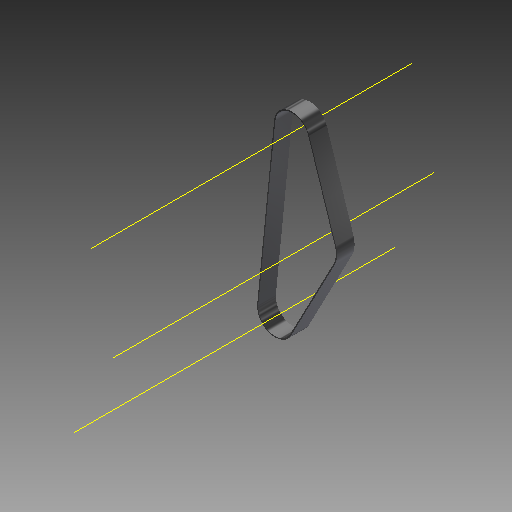
# Autodesk Inventor part: Synchronous Belt
Saved by Autodesk Inventor 2019.4 (Build 234330000, 330)
## iProperties
Created: 2020-01-06
Part Number: Synchronous Belt
Material: Rubber
Document SubType Name: Modeling
Designer: admin
Density: 1 g/cm^3
Appearance: Rubber - Black - Version 1.1
CustomPartVersion: 1
Author: admin
Autodesk Inventor part; units mm, degrees
ref_plane "YZ Plane" through (0, 0, 0) normal (1, 0, 0) x (0, 1, 0)
ref_plane "XZ Plane" through (0, 0, 0) normal (0, 1, 0) x (-1, 0, 0)
ref_plane "XY Plane" through (0, 0, 0) normal (0, 0, 1) x (1, 0, 0)
sketch "Sketch Path" plane through (0, 0, 0) normal (0, 0, 1) x (1, 0, 0)
  arc A0 (-17.1486, -148.689) -> (12.7796, -157.6858) centre (-1.314, -150.2918) ccw
  arc A1 (29.2855, 7.4127) -> (-1.6838, 4.0918) centre (14.1508, 2.489) ccw
  arc A2 (52.2256, -82.4982) -> (53.5269, -67.101) centre (34.6085, -73.2557) ccw
  line L0 (52.2256, -82.4982) -> (12.7796, -157.6858)
  line L1 (-17.1486, -148.689) -> (-1.6838, 4.0918)
  line L2 (29.2855, 7.4127) -> (53.5269, -67.101)
  constraints: 6 end point, 6 point on circle, 3 centre point
ref_plane "Cross Section Plane" through (12.7796, -157.6858, 0) normal (0.4645795, 0.8855314, 0) x (0, 0, 1)
ref_plane "Work Plane2" through (-1.314, -150.2918, 0) normal (-1, 0, 0) x (0, 0, 1)
ref_plane "Work Plane3" through (14.1508, 2.489, 0) normal (-0.3935975, -0.9192829, 0) x (0, 0, 1)
ref_plane "Work Plane4" through (34.6085, -73.2557, 0) normal (-0.1587052, 0.987326, 0) x (0, 0, 1)
sketch "Cross Section" plane through (12.7796, -157.6858, 0) normal (0.4645795, 0.8855314, 0) x (0, 0, 1)
  line L0 (-8, 0.5) -> (8, 0.5)
  line L1 (8, 0.5) -> (8, -0.5)
  line L2 (8, -0.5) -> (-8, -0.5)
  line L3 (-8, -0.5) -> (-8, 0.5)
  line L4 (-8, 0) -> (8, 0) construction
  point P0 (0, 0)
  point P1 (0, 0)
  dimension "d0" = 16
  dimension "d4" = 0.5
  dimension "d5" = 0.5
  constraints: 10 end point, 3 midpoint, 2 parallel, 1 coincident, 1 horizontal, 1 perpendicular, 1 other
  measures "d0" distance between parallel lines of L1 L3
  measures "d4" distance between parallel lines of L2 L4
  measures "d5" distance between parallel lines of L4 L0
sweep "Belt" add profiles "Cross Section" path "Sketch Path" path curves L2 A2 L0 A0 L1 A1
equation "\"d0\" = da_B"
equation "\"d4\" = da_a"
equation "\"d5\" = da_a2"
equation "\"da_B\" = 16"
equation "\"da_pb\" = 5"
equation "\"da_a\" = 0.5"
equation "\"da_S\" = 2.65"
equation "\"da_Beta\" = 20deg"
equation "\"da_Ht\" = 1.2"
equation "\"da_H\" = 2.2"
equation "\"da_a2\" = 0.5"
body "Solid1"
